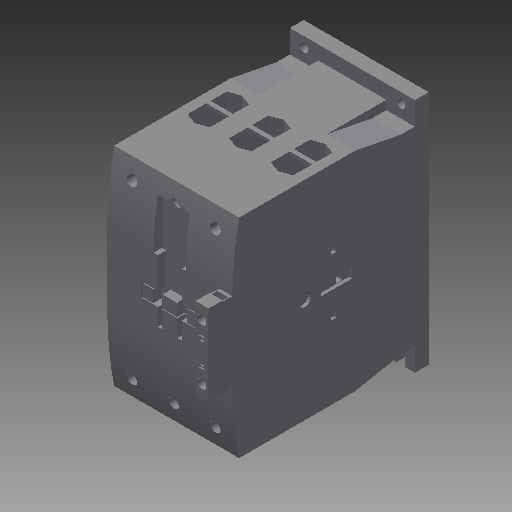
# Autodesk Inventor part: 239416
Saved by Autodesk Inventor 2019.3 (Build 233278000, 278)
## iProperties
Category: PARTsolutions
Company: MOELLER
Created: 2018-10-25
Part Number: 239416
Material: Generic
Catalog Web Link: www.cadenas.de
Description: DC operated-
Vendor: MOELLER
Document SubType Name: Modeling
Designer: psadmin
Manufacturer: MOELLER
Mass: 1810.88 g
Surface Area: 1264.18 cm^2
Volume: 1810.88 cm^3
Density: 1 g/cm^3
Appearance: PSOLRGB-175-175-175
PSOL_IDENT_0: {$CADENAS_DATA\23d-libs\moeller\2\695\733\735\737\740.prj},171 {VTYP=3D},{NB=239416},{LINA=239416},{
PSOL_IDENT_1: NN=DC operated},{DATE=04.10.2018 12:16:44},{GEOMDATE=04.10.2018 08:29:25},{VERSION=v181004082925},{L
PSOL_IDENT_2: INEID=190},{WBVAR=},{WBNUMERIC=}  {NB=239416},{LINA=239416},{KT=DUMMY},{PFOTO=2110pic-229.jpg},{PLID=
PSOL_IDENT_3: 239416},{DATA_SHEET=Data sheet},{MANUTYPEDESC=DILM80(RDC24)},{DESCSHORT=Contactor, 3p, 37kW/400V/AC3
PSOL_IDENT_4: },{DESCLONG=Contactor, Application: Contactors for Motors, Contactors up to 170 A, 3 pole, Utilizati
PSOL_IDENT_5: on category: AC-1: Non-inductive or slightly inductive loads, resistance furnaces, NAC-3: Normal AC
PSOL_IDENT_6: induction motors: starting, switch off during running, AC-4: Normal AC induction motors: starting, p
PSOL_IDENT_7: lugging, reversing, inching, Connection technique: Screw terminals, Notes: Also suitable for motors
PSOL_IDENT_8: with efficiency class IE3., IE3-ready devices are identified by the logo on their packaging., Number
PSOL_IDENT_9: of poles: 3 pole, Rated operational current AC-3 380 V 400 V: Ie= 80 A, Rated operational current A
PSOL_IDENT_10: C-1 Conventional free air thermal current, 3 pole, 50 - 60 Hz Open at 40 °C: Ith =Ie= 110 A, enclose
PSOL_IDENT_11: d: Ith= 80 A, Rated operational current AC-1 Conventional free air thermal current, 1 pole open: Ith=
PSOL_IDENT_12: 225 A, enclosed: Ith= 200 A, Max. rating for three-phase motors, 50 - 60 Hz AC-3 220 V 230 V: P= 25
PSOL_IDENT_13: kW, 380 V 400 V: P= 37 kW, 660 V 690 V: P= 63 kW, Max. rating for three-phase motors, 50 - 60 Hz AC
PSOL_IDENT_14: -4 220 V 230 V: P= 12 kW, 380 V 400 V: P= 20 kW, 660 V 690 V: P= 26 kW, Can be combined with auxilia
PSOL_IDENT_15: ry contact: DILM150-XHI(V).., DILM1000-XHI(V).., Instructions: Contacts to EN 50 012., integrated su
PSOL_IDENT_16: ppressor circuit in actuating electronics, Voltage AC/DC: DC operation},{EAN=4015082394165},{ECLASS_
PSOL_IDENT_17: 8_1=27-37-10-03},{PACKAGED_WEIGHT=2.250},{DATA_SHEET_=http://datasheet.moeller.net/datasheet.php?mod
PSOL_IDENT_18: el=239416&locale=en_GB},{DATA_SHEET_ENG=http://datasheet.moeller.net/datasheet.php?model=239416&loca
PSOL_IDENT_19: le=en_GB},{DATA_SHEET_DEU=http://datasheet.moeller.net/datasheet.php?model=239416&locale=de_DE}
NN: DC operated
NB: 239416
NBSYN: $PLID.
LINA: 239416
PFOTO: 2110pic-229.jpg
PLID: 239416
DATA_SHEET: Data sheet
MANUTYPEDESC: DILM80(RDC24)
DESCSHORT: Contactor, 3p, 37kW/400V/AC3
DESCLONG: Contactor, Application: Contactors for Motors, Contactors up to 170 A, 3 pole, Utilization category: AC-1: Non-inductive or slightly inductive loads, resistance furnaces, NAC-3: Normal AC induction motors: starting, switch off during running, AC-4: Normal AC induction motors: starting, plugging, reversing, inching, Connection technique: Screw terminals, Notes: Also suitable for motors with efficiency class IE3., IE3-ready devices are identified by the logo on their packaging., Number of poles: 3 pole, Rated operational current AC-3 380 V 400 V: Ie= 80 A, Rated operational current AC-1 Conventional free air thermal current, 3 pole, 50 - 60 Hz Open at 40 °C: Ith =Ie= 110 A, enclosed: Ith= 80 A, Rated operational current AC-1 Conventional free air thermal current, 1 pole open: Ith= 225 A, enclosed: Ith= 200 A, Max. rating for three-phase motors, 50 - 60 Hz AC-3 220 V 230 V: P= 25 kW, 380 V 400 V: P= 37 kW, 660 V 690 V: P= 63 kW, Max. rating for three-phase motors, 50 - 60 Hz AC-4 220 V 230 V: P= 12 kW, 380 V 400 V: P= 20 kW, 660 V 690 V: P= 26 kW, Can be combined with auxiliary contact: DILM150-XHI(V).., DILM1000-XHI(V).., Instructions: Contacts to EN 50 012., integrated suppressor circuit in actuating electronics, Voltage AC/DC: DC operation
EAN: 4015082394165
ECLASS_8_1: 27-37-10-03
PACKAGED_WEIGHT: 2.25
SUPPLIER: MOELLER
ARTICLENO: 239416
BOMINFO: 239416
CREATOR: CADENAS GmbH
Title: 239416
Author: Cadenas PARTsolutions
Autodesk Inventor part; units mm, degrees
sketch "Sketch_1" plane through (0, 0, 0) normal (1, 0, 0) x (0, 1, 0)
  line L0 (25.2506, 141.5) -> (-25.2506, 141.5)
  arc A0 (-25.2506, 141.5) -> (-75, 136.5) centre (-25.2506, -108.5) ccw
  line L1 (-75, 136.5) -> (-75, 52.9)
  line L2 (-75, 52.9) -> (-68.5, 20)
  line L3 (-68.5, 20) -> (-68.5, 10)
  line L4 (-68.5, 10) -> (-85, 10)
  line L5 (-85, 10) -> (-85, 0)
  line L6 (-85, 0) -> (85, 0)
  line L7 (85, 0) -> (85, 10)
  line L8 (85, 10) -> (68.5, 10)
  line L9 (68.5, 10) -> (68.5, 20)
  line L10 (68.5, 20) -> (75, 52.9)
  line L11 (75, 52.9) -> (75, 136.5)
  arc A1 (75, 136.5) -> (25.2506, 141.5) centre (25.2506, -108.5) ccw
  constraints: 24 end point, 4 point on circle, 2 centre point
extrude "Extrusion1" add sketch "Sketch_1" along normal blind 90
sketch "Sketch_2" plane through (45, 0, 0) normal (1, 0, 0) x (0, 0, -1)
  line L0 (-60, -75) -> (-10, -75)
  line L1 (-10, -75) -> (-10, 75)
  line L2 (-10, 75) -> (-60, 75)
  line L3 (-60, 75) -> (-60, -75)
  constraints: 8 end point
extrude "Extrusion2" add sketch "Sketch_2" along normal mid plane 49
sketch "Sketch_3" plane through (0, 0, 0) normal (0, 0, 1) x (1, 0, 0)
  line L0 (6.75, -78) -> (6.75, -86)
  line L1 (6.75, -86) -> (83.25, -86)
  line L2 (83.25, -86) -> (83.25, -78)
  arc A0 (83.25, -78) -> (76.75, -78) centre (80, -78) ccw
  line L3 (76.75, -78) -> (76.75, -85.5)
  line L4 (76.75, -85.5) -> (13.25, -85.5)
  line L5 (13.25, -85.5) -> (13.25, -78)
  arc A1 (13.25, -78) -> (6.75, -78) centre (10, -78) ccw
  constraints: 12 end point, 4 point on circle, 2 centre point
extrude "Extrusion3" cut sketch "Sketch_3" along normal blind 10
sketch "Sketch4" plane through (0, -85, 0) normal (0, 0, -1) x (-1, 0, 0)
  point P0 (-10, 163)
hole "Hole1" at (10, 78, 0) direction (0, 0, 1) diameter 6.5 depth 10
sketch "Sketch5" plane through (0, -85, 0) normal (0, 0, -1) x (-1, 0, 0)
  point P0 (-80, 163)
hole "Hole2" at (80, 78, 0) direction (0, 0, 1) diameter 6.5 depth 10
sketch "Sketch_6" plane through (12, 0, 0) normal (1, 0, 0) x (0, 0, -1)
  line L0 (0, 61.5) -> (-35.9, 61.5)
  line L1 (-35.9, 61.5) -> (-35.9, 66)
  line L2 (-35.9, 66) -> (0, 66.6266)
  line L3 (0, 66.6266) -> (0, 61.5)
  line L4 (0, 61.5) -> (-35.9, 61.5)
  constraints: 10 end point
revolve "Revolution1" cut sketch "Sketch_6" angle 360 about axis through (12, 61.5, 0) along (0, 0, -1)
sketch "Sketch_7" plane through (12, 0, 0) normal (1, 0, 0) x (0, 0, -1)
  line L0 (0, -61.5) -> (-35.9, -61.5)
  line L1 (-35.9, -61.5) -> (-35.9, -57)
  line L2 (-35.9, -57) -> (0, -56.3734)
  line L3 (0, -56.3734) -> (0, -61.5)
  line L4 (0, -61.5) -> (-35.9, -61.5)
  constraints: 10 end point
revolve "Revolution2" cut sketch "Sketch_7" angle 360 about axis through (12, -61.5, 0) along (0, 0, -1)
sketch "Sketch_8" plane through (78, 0, 0) normal (1, 0, 0) x (0, 0, -1)
  line L0 (0, 61.5) -> (-35.9, 61.5)
  line L1 (-35.9, 61.5) -> (-35.9, 66)
  line L2 (-35.9, 66) -> (0, 66.6266)
  line L3 (0, 66.6266) -> (0, 61.5)
  line L4 (0, 61.5) -> (-35.9, 61.5)
  constraints: 10 end point
revolve "Revolution3" cut sketch "Sketch_8" angle 360 about axis through (78, 61.5, 0) along (0, 0, -1)
sketch "Sketch_9" plane through (78, 0, 0) normal (1, 0, 0) x (0, 0, -1)
  line L0 (0, -61.5) -> (-35.9, -61.5)
  line L1 (-35.9, -61.5) -> (-35.9, -57)
  line L2 (-35.9, -57) -> (0, -56.3734)
  line L3 (0, -56.3734) -> (0, -61.5)
  line L4 (0, -61.5) -> (-35.9, -61.5)
  constraints: 10 end point
revolve "Revolution4" cut sketch "Sketch_9" angle 360 about axis through (78, -61.5, 0) along (0, 0, -1)
sketch "Sketch_10" plane through (0, 0, 0) normal (0, 1, 0) x (-1, 0, 0)
  line L0 (-6.9, 62.4482) -> (-6.9, 74)
  line L1 (-6.9, 74) -> (-23.1, 74)
  line L2 (-23.1, 74) -> (-23.1, 62.4482)
  line L3 (-23.1, 62.4482) -> (-15, 59.5)
  line L4 (-15, 59.5) -> (-6.9, 62.4482)
  constraints: 10 end point
extrude "Extrusion4" cut sketch "Sketch_10" along normal mid plane 200
sketch "Sketch_11" plane through (0, 0, 0) normal (0, 1, 0) x (-1, 0, 0)
  line L0 (-36.9, 62.4482) -> (-36.9, 74)
  line L1 (-36.9, 74) -> (-53.1, 74)
  line L2 (-53.1, 74) -> (-53.1, 62.4482)
  line L3 (-53.1, 62.4482) -> (-45, 59.5)
  line L4 (-45, 59.5) -> (-36.9, 62.4482)
  constraints: 10 end point
extrude "Extrusion5" cut sketch "Sketch_11" along normal mid plane 200
sketch "Sketch_12" plane through (0, 0, 0) normal (0, 1, 0) x (-1, 0, 0)
  line L0 (-66.9, 62.4482) -> (-66.9, 74)
  line L1 (-66.9, 74) -> (-83.1, 74)
  line L2 (-83.1, 74) -> (-83.1, 62.4482)
  line L3 (-83.1, 62.4482) -> (-75, 59.5)
  line L4 (-75, 59.5) -> (-66.9, 62.4482)
  constraints: 10 end point
extrude "Extrusion6" cut sketch "Sketch_12" along normal mid plane 200
sketch "Sketch_13" plane through (0, 0, 0) normal (0, 1, 0) x (-1, 0, 0)
  line L0 (-6.9, 90.6518) -> (-15, 93.6)
  line L1 (-15, 93.6) -> (-23.1, 90.6518)
  line L2 (-23.1, 90.6518) -> (-23.1, 77)
  line L3 (-23.1, 77) -> (-6.9, 77)
  line L4 (-6.9, 77) -> (-6.9, 90.6518)
  constraints: 10 end point
extrude "Extrusion7" cut sketch "Sketch_13" along normal mid plane 200
sketch "Sketch_14" plane through (0, 0, 0) normal (0, 1, 0) x (-1, 0, 0)
  line L0 (-36.9, 90.6518) -> (-45, 93.6)
  line L1 (-45, 93.6) -> (-53.1, 90.6518)
  line L2 (-53.1, 90.6518) -> (-53.1, 77)
  line L3 (-53.1, 77) -> (-36.9, 77)
  line L4 (-36.9, 77) -> (-36.9, 90.6518)
  constraints: 10 end point
extrude "Extrusion8" cut sketch "Sketch_14" along normal mid plane 200
sketch "Sketch_15" plane through (0, 0, 0) normal (0, 1, 0) x (-1, 0, 0)
  line L0 (-66.9, 90.6518) -> (-75, 93.6)
  line L1 (-75, 93.6) -> (-83.1, 90.6518)
  line L2 (-83.1, 90.6518) -> (-83.1, 77)
  line L3 (-83.1, 77) -> (-66.9, 77)
  line L4 (-66.9, 77) -> (-66.9, 90.6518)
  constraints: 10 end point
extrude "Extrusion9" cut sketch "Sketch_15" along normal mid plane 200
sketch "Sketch_16" plane through (0, 0, 0) normal (0, 1, 0) x (-1, 0, 0)
  line L0 (-2, 100) -> (-88, 100)
  line L1 (-88, 100) -> (-88, 50)
  line L2 (-88, 50) -> (-2, 50)
  line L3 (-2, 50) -> (-2, 100)
  constraints: 8 end point
extrude "Extrusion10" add sketch "Sketch_16" along normal mid plane 104
sketch "Sketch_17" plane through (45, 0, 0) normal (1, 0, 0) x (0, 0, -1)
  arc A0 (-93.1, -0.5) -> (-84.9, -0.5) centre (-89, -0.5) ccw
  line L0 (-84.9, -0.5) -> (-84.9, 0.5)
  arc A1 (-84.9, 0.5) -> (-93.1, 0.5) centre (-89, 0.5) ccw
  line L1 (-93.1, 0.5) -> (-93.1, -0.5)
  constraints: 4 end point, 4 point on circle, 2 centre point
extrude "Extrusion11" cut sketch "Sketch_17" along normal mid plane 146
sketch "Sketch_19" plane through (45, 0, 0) normal (1, 0, 0) x (0, 0, -1)
  line L0 (-77.9, -3.6) -> (-55.3, -3.6)
  line L1 (-55.3, -3.6) -> (-55.3, 3.6)
  line L2 (-55.3, 3.6) -> (-77.9, 3.6)
  line L3 (-77.9, 3.6) -> (-77.9, -3.6)
  constraints: 8 end point
extrude "Extrusion12" cut sketch "Sketch_19" along normal mid plane 100
sketch "Sketch_18" plane through (45, 0, 0) normal (1, 0, 0) x (0, 0, -1)
  line L0 (-100, -10) -> (-50, -10)
  line L1 (-50, -10) -> (-50, 10)
  line L2 (-50, 10) -> (-100, 10)
  line L3 (-100, 10) -> (-100, -10)
  line L4 (-64.4, -3.2) -> (-60.1, -3.2)
  line L5 (-60.1, -3.2) -> (-60.1, 3.2)
  line L6 (-60.1, 3.2) -> (-64.4, 3.2)
  line L7 (-64.4, 3.2) -> (-64.4, -3.2)
  constraints: 16 end point
extrude "Extrusion13" add sketch "Sketch_18" along normal mid plane 85.6
sketch "Sketch_20" plane through (90, 0, 0) normal (1, 0, 0) x (0, 0, -1)
  line L0 (-158.8, 15) -> (-158.8, -15)
  arc A0 (-158.8, -15) -> (-158.5505, -29.3) centre (251.2, -15) ccw
  line L1 (-158.5505, -29.3) -> (-148.4, -29.3)
  line L2 (-148.4, -29.3) -> (-148.4, -28.5)
  line L3 (-148.4, -28.5) -> (-128.8, -28.5)
  line L4 (-128.8, -28.5) -> (-128.8, 28.5)
  line L5 (-128.8, 28.5) -> (-148.4, 28.5)
  line L6 (-148.4, 28.5) -> (-148.4, 29.3)
  line L7 (-148.4, 29.3) -> (-158.5505, 29.3)
  arc A1 (-158.5505, 29.3) -> (-158.8, 15) centre (251.2, 15) ccw
  constraints: 16 end point, 4 point on circle, 2 centre point
extrude "Extrusion14" add sketch "Sketch_20" against normal blind 9.4
sketch "Sketch_21" plane through (45, 0, 0) normal (1, 0, 0) x (0, 0, -1)
  line L0 (-70.7, 18.9) -> (-66.7, 18.9)
  line L1 (-66.7, 18.9) -> (-66.7, 22.4)
  line L2 (-66.7, 22.4) -> (-70.7, 22.4)
  line L3 (-70.7, 22.4) -> (-70.7, 18.9)
  constraints: 8 end point
extrude "Extrusion15" cut sketch "Sketch_21" along normal mid plane 100
sketch "Sketch_22" plane through (45, 0, 0) normal (1, 0, 0) x (0, 0, -1)
  line L0 (-70.7, -18.9) -> (-70.7, -22.4)
  line L1 (-70.7, -22.4) -> (-66.7, -22.4)
  line L2 (-66.7, -22.4) -> (-66.7, -18.9)
  line L3 (-66.7, -18.9) -> (-70.7, -18.9)
  constraints: 8 end point
extrude "Extrusion16" cut sketch "Sketch_22" along normal mid plane 100
sketch "Sketch_23" plane through (45, 0, 0) normal (1, 0, 0) x (0, 0, -1)
  line L0 (-80, -17.4) -> (-80, -22.4)
  line L1 (-80, -22.4) -> (-50, -22.4)
  line L2 (-50, -22.4) -> (-50, 22.4)
  line L3 (-50, 22.4) -> (-80, 22.4)
  line L4 (-80, 22.4) -> (-80, 17.4)
  line L5 (-80, 17.4) -> (-55, 17.4)
  line L6 (-55, 17.4) -> (-55, -17.4)
  line L7 (-55, -17.4) -> (-80, -17.4)
  constraints: 16 end point
extrude "Extrusion17" add sketch "Sketch_23" along normal mid plane 86
sketch "Sketch_24" plane through (0, 0, 141.5) normal (0, 0, 1) x (1, 0, 0)
  line L0 (24.6, 5) -> (24.6, -5)
  line L1 (24.6, -5) -> (65.4, -5)
  line L2 (65.4, -5) -> (65.4, 5)
  line L3 (65.4, 5) -> (53.5, 5)
  line L4 (53.5, 5) -> (53.5, 27.4308)
  line L5 (53.5, 27.4308) -> (56.5, 27.4308)
  line L6 (56.5, 27.4308) -> (56.5, 62.3)
  line L7 (56.5, 62.3) -> (33.5, 62.3)
  line L8 (33.5, 62.3) -> (33.5, 27.4308)
  line L9 (33.5, 27.4308) -> (36.5, 27.4308)
  line L10 (36.5, 27.4308) -> (36.5, 5)
  line L11 (36.5, 5) -> (24.6, 5)
  line L12 (57.1, -4.45) -> (64.5, -4.45)
  line L13 (64.5, -4.45) -> (64.5, 4.45)
  line L14 (64.5, 4.45) -> (57.1, 4.45)
  line L15 (57.1, 4.45) -> (57.1, -4.45)
  line L16 (39.75, 4.45) -> (39.75, -4.45)
  line L17 (39.75, -4.45) -> (50.25, -4.45)
  line L18 (50.25, -4.45) -> (50.25, 4.45)
  line L19 (50.25, 4.45) -> (39.75, 4.45)
  line L20 (25.5, -4.45) -> (32.9, -4.45)
  line L21 (32.9, -4.45) -> (32.9, 4.45)
  line L22 (32.9, 4.45) -> (25.5, 4.45)
  line L23 (25.5, 4.45) -> (25.5, -4.45)
  constraints: 48 end point
extrude "Extrusion18" cut sketch "Sketch_24" against normal blind 6
sketch "Sketch_25" plane through (0, 0, 141.5) normal (0, 0, 1) x (1, 0, 0)
  line L0 (36.5, -4.6) -> (36.5, -17.3)
  line L1 (36.5, -17.3) -> (39.5, -17.3)
  line L2 (39.5, -17.3) -> (39.5, -4.8)
  line L3 (39.5, -4.8) -> (50.5, -4.8)
  line L4 (50.5, -4.8) -> (50.5, -17.3)
  line L5 (50.5, -17.3) -> (53.5, -17.3)
  line L6 (53.5, -17.3) -> (53.5, -4.6)
  line L7 (53.5, -4.6) -> (36.5, -4.6)
  constraints: 16 end point
extrude "Extrusion19" cut sketch "Sketch_25" against normal blind 5.5
sketch "Sketch_26" plane through (0, 0, 141.5) normal (0, 0, 1) x (1, 0, 0)
  circle A0 centre (15, 61.95) radius 3.85
  constraints: 1 centre point
extrude "Extrusion20" cut sketch "Sketch_26" against normal blind 13.9
sketch "Sketch_27" plane through (0, 0, 141.5) normal (0, 0, 1) x (1, 0, 0)
  circle A0 centre (45, 61.95) radius 3.85
  constraints: 1 centre point
extrude "Extrusion21" cut sketch "Sketch_27" against normal blind 13.9
sketch "Sketch_28" plane through (0, 0, 141.5) normal (0, 0, 1) x (1, 0, 0)
  circle A0 centre (75, 61.95) radius 3.85
  constraints: 1 centre point
extrude "Extrusion22" cut sketch "Sketch_28" against normal blind 13.9
sketch "Sketch_29" plane through (0, 0, 141.5) normal (0, 0, 1) x (1, 0, 0)
  circle A0 centre (15, -61.95) radius 3.85
  constraints: 1 centre point
extrude "Extrusion23" cut sketch "Sketch_29" against normal blind 13.9
sketch "Sketch_30" plane through (0, 0, 141.5) normal (0, 0, 1) x (1, 0, 0)
  circle A0 centre (45, -61.95) radius 3.85
  constraints: 1 centre point
extrude "Extrusion24" cut sketch "Sketch_30" against normal blind 13.9
sketch "Sketch_31" plane through (0, 0, 141.5) normal (0, 0, 1) x (1, 0, 0)
  circle A0 centre (75, -61.95) radius 3.85
  constraints: 1 centre point
extrude "Extrusion25" cut sketch "Sketch_31" against normal blind 13.9
sketch "Sketch_32" plane through (0, 0, 141.5) normal (0, 0, 1) x (1, 0, 0)
  line L0 (12.5, 60.5066) -> (15, 59.0632)
  line L1 (15, 59.0632) -> (17.5, 60.5066)
  line L2 (17.5, 60.5066) -> (17.5, 63.3934)
  line L3 (17.5, 63.3934) -> (15, 64.8368)
  line L4 (15, 64.8368) -> (12.5, 63.3934)
  line L5 (12.5, 63.3934) -> (12.5, 60.5066)
  constraints: 12 end point
extrude "Extrusion26" cut sketch "Sketch_32" against normal blind 17.9
sketch "Sketch_33" plane through (0, 0, 141.5) normal (0, 0, 1) x (1, 0, 0)
  line L0 (42.5, 60.5066) -> (45, 59.0632)
  line L1 (45, 59.0632) -> (47.5, 60.5066)
  line L2 (47.5, 60.5066) -> (47.5, 63.3934)
  line L3 (47.5, 63.3934) -> (45, 64.8368)
  line L4 (45, 64.8368) -> (42.5, 63.3934)
  line L5 (42.5, 63.3934) -> (42.5, 60.5066)
  constraints: 12 end point
extrude "Extrusion27" cut sketch "Sketch_33" against normal blind 17.9
sketch "Sketch_34" plane through (0, 0, 141.5) normal (0, 0, 1) x (1, 0, 0)
  line L0 (72.5, 60.5066) -> (75, 59.0632)
  line L1 (75, 59.0632) -> (77.5, 60.5066)
  line L2 (77.5, 60.5066) -> (77.5, 63.3934)
  line L3 (77.5, 63.3934) -> (75, 64.8368)
  line L4 (75, 64.8368) -> (72.5, 63.3934)
  line L5 (72.5, 63.3934) -> (72.5, 60.5066)
  constraints: 12 end point
extrude "Extrusion28" cut sketch "Sketch_34" against normal blind 17.9
sketch "Sketch_35" plane through (0, 0, 141.5) normal (0, 0, 1) x (1, 0, 0)
  line L0 (12.5, -63.3934) -> (15, -64.8368)
  line L1 (15, -64.8368) -> (17.5, -63.3934)
  line L2 (17.5, -63.3934) -> (17.5, -60.5066)
  line L3 (17.5, -60.5066) -> (15, -59.0632)
  line L4 (15, -59.0632) -> (12.5, -60.5066)
  line L5 (12.5, -60.5066) -> (12.5, -63.3934)
  constraints: 12 end point
extrude "Extrusion29" cut sketch "Sketch_35" against normal blind 17.9
sketch "Sketch_36" plane through (0, 0, 141.5) normal (0, 0, 1) x (1, 0, 0)
  line L0 (42.5, -63.3934) -> (45, -64.8368)
  line L1 (45, -64.8368) -> (47.5, -63.3934)
  line L2 (47.5, -63.3934) -> (47.5, -60.5066)
  line L3 (47.5, -60.5066) -> (45, -59.0632)
  line L4 (45, -59.0632) -> (42.5, -60.5066)
  line L5 (42.5, -60.5066) -> (42.5, -63.3934)
  constraints: 12 end point
extrude "Extrusion30" cut sketch "Sketch_36" against normal blind 17.9
sketch "Sketch_37" plane through (0, 0, 141.5) normal (0, 0, 1) x (1, 0, 0)
  line L0 (72.5, -63.3934) -> (75, -64.8368)
  line L1 (75, -64.8368) -> (77.5, -63.3934)
  line L2 (77.5, -63.3934) -> (77.5, -60.5066)
  line L3 (77.5, -60.5066) -> (75, -59.0632)
  line L4 (75, -59.0632) -> (72.5, -60.5066)
  line L5 (72.5, -60.5066) -> (72.5, -63.3934)
  constraints: 12 end point
extrude "Extrusion31" cut sketch "Sketch_37" against normal blind 17.9
sketch "Sketch_38" plane through (0, 0, 158.8) normal (0, 0, 1) x (1, 0, 0)
  line L0 (83.4309, 9.3809) -> (87.1691, 9.3809)
  line L1 (87.1691, 9.3809) -> (87.1691, 10.6191)
  line L2 (87.1691, 10.6191) -> (83.4309, 10.6191)
  line L3 (83.4309, 10.6191) -> (83.4309, 9.3809)
  constraints: 8 end point
extrude "Extrusion32" cut sketch "Sketch_38" against normal blind 1.05
sketch "Sketch_39" plane through (0, 0, 158.8) normal (0, 0, 1) x (1, 0, 0)
  line L0 (84, 6.7) -> (87, 6.7)
  line L1 (87, 6.7) -> (87, 8.4)
  line L2 (87, 8.4) -> (84, 8.4)
  line L3 (84, 8.4) -> (84, 6.7)
  constraints: 8 end point
extrude "Extrusion33" cut sketch "Sketch_39" against normal blind 1.05
sketch "Sketch40" plane through (90, -15, 158.8) normal (0, 0, 1) x (1, 0, 0)
  point P0 (-4.5, 7.7)
hole "Hole3" at (85.5, -7.3, 158.8) direction (0, 0, -1) diameter 3.18 depth 1.05
sketch "Sketch_41" plane through (0, 0, 158.8) normal (0, 0, 1) x (1, 0, 0)
  line L0 (83.4309, -10.6191) -> (87.1691, -10.6191)
  line L1 (87.1691, -10.6191) -> (87.1691, -9.3809)
  line L2 (87.1691, -9.3809) -> (83.4309, -9.3809)
  line L3 (83.4309, -9.3809) -> (83.4309, -10.6191)
  constraints: 8 end point
extrude "Extrusion34" cut sketch "Sketch_41" against normal blind 1.05
sketch "Sketch_42" plane through (0, 0, 0) normal (0, 1, 0) x (-1, 0, 0)
  line L0 (-81.4, 148.4) -> (-89.2, 148.4)
  line L1 (-89.2, 148.4) -> (-89.2, 143.7)
  line L2 (-89.2, 143.7) -> (-81.4, 143.7)
  line L3 (-81.4, 143.7) -> (-81.4, 148.4)
  constraints: 8 end point
extrude "Extrusion35" cut sketch "Sketch_42" along normal mid plane 100
sketch "Sketch_43" plane through (0, 0, 0) normal (0, 1, 0) x (-1, 0, 0)
  line L0 (-81.4, 148.4) -> (-89.2, 148.4)
  line L1 (-89.2, 148.4) -> (-89.2, 143.7)
  line L2 (-89.2, 143.7) -> (-81.4, 143.7)
  line L3 (-81.4, 143.7) -> (-81.4, 148.4)
  constraints: 8 end point
extrude "Extrusion36" add sketch "Sketch_43" along normal mid plane 29.9
sketch "Sketch_44" plane through (85.3, 0, 0) normal (1, 0, 0) x (0, 0, -1)
  line L0 (-137.85, 20) -> (-148.95, 20)
  line L1 (-148.95, 20) -> (-148.95, 23)
  line L2 (-148.95, 23) -> (-146.55, 23)
  line L3 (-146.55, 23) -> (-146.55, 21.75)
  line L4 (-146.55, 21.75) -> (-137.85, 21.75)
  line L5 (-137.85, 21.75) -> (-137.85, 20)
  line L6 (-137.85, 20) -> (-148.95, 20)
  constraints: 14 end point
revolve "Revolution5" add sketch "Sketch_44" angle 360 about axis through (85.3, 20, 137.85) along (0, 0, -1)
sketch "Sketch_45" plane through (85.3, 0, 0) normal (1, 0, 0) x (0, 0, -1)
  line L0 (-137.85, -20) -> (-148.95, -20)
  line L1 (-148.95, -20) -> (-148.95, -17)
  line L2 (-148.95, -17) -> (-146.55, -17)
  line L3 (-146.55, -17) -> (-146.55, -18.25)
  line L4 (-146.55, -18.25) -> (-137.85, -18.25)
  line L5 (-137.85, -18.25) -> (-137.85, -20)
  line L6 (-137.85, -20) -> (-148.95, -20)
  constraints: 14 end point
revolve "Revolution6" add sketch "Sketch_45" angle 360 about axis through (85.3, -20, 137.85) along (0, 0, -1)
sketch "Sketch_46" plane through (0, 0, 74) normal (0, 0, 1) x (1, 0, 0)
  line L0 (6.9, 52) -> (23.1, 52)
  line L1 (23.1, 52) -> (23.1, 73)
  line L2 (23.1, 73) -> (6.9, 73)
  line L3 (6.9, 73) -> (6.9, 52)
  constraints: 8 end point
extrude "Extrusion37" cut sketch "Sketch_46" along normal blind 10
sketch "Sketch_47" plane through (0, 0, 74) normal (0, 0, 1) x (1, 0, 0)
  line L0 (36.9, 52) -> (53.1, 52)
  line L1 (53.1, 52) -> (53.1, 73)
  line L2 (53.1, 73) -> (36.9, 73)
  line L3 (36.9, 73) -> (36.9, 52)
  constraints: 8 end point
extrude "Extrusion38" cut sketch "Sketch_47" along normal blind 10
sketch "Sketch_48" plane through (0, 0, 74) normal (0, 0, 1) x (1, 0, 0)
  line L0 (66.9, 52) -> (83.1, 52)
  line L1 (83.1, 52) -> (83.1, 73)
  line L2 (83.1, 73) -> (66.9, 73)
  line L3 (66.9, 73) -> (66.9, 52)
  constraints: 8 end point
extrude "Extrusion39" cut sketch "Sketch_48" along normal blind 10
sketch "Sketch_49" plane through (0, 0, 74) normal (0, 0, 1) x (1, 0, 0)
  line L0 (6.9, -52) -> (6.9, -73)
  line L1 (6.9, -73) -> (23.1, -73)
  line L2 (23.1, -73) -> (23.1, -52)
  line L3 (23.1, -52) -> (6.9, -52)
  constraints: 8 end point
extrude "Extrusion40" cut sketch "Sketch_49" along normal blind 10
sketch "Sketch_50" plane through (0, 0, 74) normal (0, 0, 1) x (1, 0, 0)
  line L0 (36.9, -52) -> (36.9, -73)
  line L1 (36.9, -73) -> (53.1, -73)
  line L2 (53.1, -73) -> (53.1, -52)
  line L3 (53.1, -52) -> (36.9, -52)
  constraints: 8 end point
extrude "Extrusion41" cut sketch "Sketch_50" along normal blind 10
sketch "Sketch_51" plane through (0, 0, 74) normal (0, 0, 1) x (1, 0, 0)
  line L0 (66.9, -52) -> (66.9, -73)
  line L1 (66.9, -73) -> (83.1, -73)
  line L2 (83.1, -73) -> (83.1, -52)
  line L3 (83.1, -52) -> (66.9, -52)
  constraints: 8 end point
extrude "Extrusion42" cut sketch "Sketch_51" along normal blind 10
sketch "Sketch_52" plane through (0, 0, 158.8) normal (0, 0, 1) x (1, 0, 0)
  circle A0 centre (85.3, 20) radius 3.3
  constraints: 1 centre point
extrude "Extrusion43" cut sketch "Sketch_52" against normal blind 9.85
sketch "Sketch_53" plane through (0, 0, 158.8) normal (0, 0, 1) x (1, 0, 0)
  circle A0 centre (85.3, -20) radius 3.3
  constraints: 1 centre point
extrude "Extrusion44" cut sketch "Sketch_53" against normal blind 9.85
sketch "Sketch_54" plane through (0, 0, 158.8) normal (0, 0, 1) x (1, 0, 0)
  line L0 (82.3951, 19.5) -> (84.8, 19.5)
  line L1 (84.8, 19.5) -> (84.8, 17.8832)
  line L2 (84.8, 17.8832) -> (85.8, 17.8832)
  line L3 (85.8, 17.8832) -> (85.8, 19.5)
  line L4 (85.8, 19.5) -> (88.2049, 19.5)
  line L5 (88.2049, 19.5) -> (88.2049, 20.5)
  line L6 (88.2049, 20.5) -> (85.8, 20.5)
  line L7 (85.8, 20.5) -> (85.8, 22.1167)
  line L8 (85.8, 22.1167) -> (84.8, 22.1167)
  line L9 (84.8, 22.1167) -> (84.8, 20.5)
  line L10 (84.8, 20.5) -> (82.3951, 20.5)
  line L11 (82.3951, 20.5) -> (82.3951, 19.5)
  constraints: 24 end point
extrude "Extrusion45" cut sketch "Sketch_54" against normal blind 11.05
sketch "Sketch_55" plane through (0, 0, 158.8) normal (0, 0, 1) x (1, 0, 0)
  line L0 (82.3951, -19.5) -> (82.3951, -20.5)
  line L1 (82.3951, -20.5) -> (84.8, -20.5)
  line L2 (84.8, -20.5) -> (84.8, -22.1167)
  line L3 (84.8, -22.1167) -> (85.8, -22.1167)
  line L4 (85.8, -22.1167) -> (85.8, -20.5)
  line L5 (85.8, -20.5) -> (88.2049, -20.5)
  line L6 (88.2049, -20.5) -> (88.2049, -19.5)
  line L7 (88.2049, -19.5) -> (85.8, -19.5)
  line L8 (85.8, -19.5) -> (85.8, -17.8832)
  line L9 (85.8, -17.8832) -> (84.8, -17.8832)
  line L10 (84.8, -17.8832) -> (84.8, -19.5)
  line L11 (84.8, -19.5) -> (82.3951, -19.5)
  constraints: 24 end point
extrude "Extrusion46" cut sketch "Sketch_55" against normal blind 11.05
ref_plane "1_XY" through (0, 0, 0) normal (0, 0, 1) x (1, 0, 0)
ref_plane "1_YZ" through (0, 0, 0) normal (1, 0, 0) x (0, 1, 0)
ref_plane "1_ZX" through (0, 0, 0) normal (0, 1, 0) x (0, 0, 1)
ref_plane "XHI_XY" through (45, 0, 141.5) normal (0, 0, -1) x (1, 0, 0)
ref_plane "XHI_YZ" through (45, 0, 141.5) normal (1, 0, 0) x (0, -1, 0)
ref_plane "XHI_ZX" through (45, 0, 141.5) normal (0, -1, 0) x (0, 0, -1)
ref_plane "XHI11_S_1_XY" through (0, 20.65, 68.7) normal (-1, 0, 0) x (0, 0, -1)
ref_plane "XHI11_S_1_YZ" through (0, 20.65, 68.7) normal (0, 0, -1) x (0, -1, 0)
ref_plane "XHI11_S_1_ZX" through (0, 20.65, 68.7) normal (0, -1, 0) x (-1, 0, 0)
ref_plane "XHI11_S_2_XY" through (90, -20.65, 68.7) normal (1, 0, 0) x (0, 0, -1)
ref_plane "XHI11_S_2_YZ" through (90, -20.65, 68.7) normal (0, 0, -1) x (0, 1, 0)
ref_plane "XHI11_S_2_ZX" through (90, -20.65, 68.7) normal (0, 1, 0) x (1, 0, 0)
ref_plane "XMV_XY" through (90, 0, 89) normal (1, 0, 0) x (0, 0, -1)
ref_plane "XMV_YZ" through (90, 0, 89) normal (0, 0, -1) x (0, 1, 0)
ref_plane "XMV_ZX" through (90, 0, 89) normal (0, 1, 0) x (1, 0, 0)
ref_plane "XSP_XY" through (90, 0, 158.8) normal (1, 0, 0) x (0, 0, -1)
ref_plane "XSP_YZ" through (90, 0, 158.8) normal (0, 0, -1) x (0, 1, 0)
ref_plane "XSP_ZX" through (90, 0, 158.8) normal (0, 1, 0) x (1, 0, 0)
body "Solid1"
